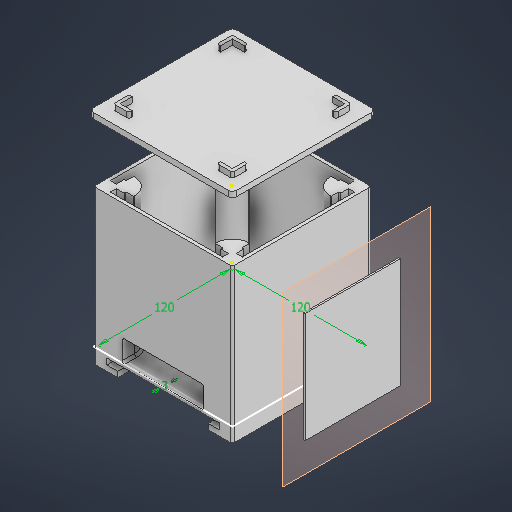
# Autodesk Inventor part: Chink_Box_FINAL
Saved by Autodesk Inventor 2026.1 (Build 301233020, 233B)
## iProperties
Created: 2026-09-22
Part Number: Chink_Box_FINAL
Material: Generic
Document SubType Name: Modeling
Designer: uali517
Density: 1 g/cm^3
Appearance: Default
Author: uali517
Autodesk Inventor part; units mm, degrees
ref_plane "YZ Plane" through (0, 0, 0) normal (1, 0, 0) x (0, 1, 0)
ref_plane "XY Plane" through (0, 0, 0) normal (0, 0, 1) x (1, 0, 0)
sketch "Sketch1" plane through (0, 0, 0) normal (0, 1, 0) x (-1, 0, 0)
  line L0 (0, 0) -> (120, 0)
  line L1 (120, 0) -> (120, -120)
  line L2 (120, -120) -> (0, -120)
  line L3 (0, -120) -> (0, 0)
  line L4 (123, 3) -> (-3, 3)
  line L5 (-3, 3) -> (-3, -123)
  line L6 (-3, -123) -> (123, -123)
  line L7 (123, -123) -> (123, 3)
  dimension "d0" = 120
  dimension "d1" = 120
  dimension "d2" = 3
  constraints: 16 end point, 4 parallel, 2 perpendicular, 1 horizontal, 3 other
  measures "d0" distance of L1.end L2.end
  measures "d1" distance of L0.end L1.end
  measures "d2" distance between parallel lines of L0 L4
extrude "Extrusion1" add sketch "Sketch1" along normal blind 126
sketch "Sketch2" plane through (0, 0, 0) normal (0, 1, 0) x (-1, 0, 0)
  line L0 (0, 0) -> (120, 0) projected
  line L1 (120, 0) -> (111, 0)
  line L2 (111, 0) -> (111, -9)
  line L3 (111, -9) -> (120, -9)
  line L4 (120, -9) -> (120, 0)
  line L5 (114.5, -5.5) -> (104, -5.5)
  line L6 (114.5, -16) -> (114.5, -5.5)
  line L7 (104, -5.5) -> (104, -16)
  line L8 (104, -16) -> (114.5, -16)
  line L9 (104, -7.3) -> (97, -7.3)
  line L10 (104, -13.4046) -> (104, -7.3)
  line L11 (112.7, -16) -> (106.6771, -16)
  line L12 (112.7, -23) -> (112.7, -16)
  line L13 (97, -7.3) -> (97, -8)
  line L14 (112, -23) -> (112.7, -23)
  arc A0 (97, -8) -> (112, -23) centre (112, -8) ccw
  point P0 (120, -120)
  point P1 (111, 0)
  point P2 (60, -60)
  point P3 (114.5, -9)
  point P4 (111, -5.5)
  dimension "d9" = 9
  dimension "d10" = 9
  dimension "d15" = 5.5
  dimension "d37" = 1.8
  dimension "d39" = 1.8
  dimension "d40" = 15
  dimension "d41" = 7
  dimension "d42" = 7
  constraints: 28 end point, 5 perpendicular, 4 horizontal, 2 parallel, 2 point on circle, 2 point on line, 2 tangent, 2 vertical, 1 centre point
  measures "d9" distance of L3.end L2.end
  measures "d10" distance of L2.end L1.end
  measures "d15" distance between parallel lines of L0 L5
  measures "d37" distance between parallel lines of L5 L9
  measures "d39" distance between parallel lines of L6 L12
  measures "d40" radius of A0
  measures "d41" distance of L9.start L9.end
  measures "d42" distance between parallel lines of L7 L2
extrude "Extrusion3" add sketch "Sketch2" along normal up to surface (126 mm away)
pattern_circular "Circular Pattern1" count 4 over 360 about axis through (-60, 0, -60) along (0, 1, 0) of "Extrusion3"
sketch "Sketch9" plane through (0, 0, 0) normal (0, 1, 0) x (-1, 0, 0)
  line L0 (97, -7.3) -> (104, -7.3) projected
  line L1 (104, -7.3) -> (104, -5.5) projected
  line L2 (104, -5.5) -> (111, -5.5) projected
  line L3 (111, -5.5) -> (111, 0) projected
  line L4 (114.5, -9) -> (114.5, -16) projected
  line L5 (112.7, -16) -> (112.7, -23) projected
  line L6 (120, -9) -> (114.5, -9) projected
  line L7 (112.7, -97) -> (112.7, -104) projected
  line L8 (112.7, -104) -> (114.5, -104) projected
  line L9 (114.5, -104) -> (114.5, -111) projected
  line L10 (114.5, -111) -> (120, -111) projected
  line L11 (9, 0) -> (9, -5.5) projected
  line L12 (9, -5.5) -> (16, -5.5) projected
  line L13 (16, -5.5) -> (16, -7.3) projected
  line L14 (16, -7.3) -> (23, -7.3) projected
  line L15 (9, 0) -> (111, 0) projected
  line L16 (120, -9) -> (120, -111) projected
  line L17 (23, -7.3) -> (23, 0)
  line L18 (97, -7.3) -> (97, 0)
  line L19 (112.7, -97) -> (120, -97)
  line L20 (112.7, -23) -> (120, -23)
  line L21 (114.5, -16) -> (112.7, -16) projected
  point P0 (0, 0)
  constraints: 8 end point, 4 point on line, 3 perpendicular, 1 vertical
extrude "Extrusion8" add sketch "Sketch9" along normal blind 20
sketch "Sketch10" plane through (-123, 0, 3) normal (0, 0, 1) x (1, 0, 0)
  line L0 (19, 20) -> (26, 20) projected
  line L1 (100, 0) -> (100, 126) projected
  line L2 (26, 20) -> (100, 20)
  line L3 (100, 20) -> (100, 0)
  line L4 (100, 0) -> (26, 0)
  line L5 (26, 0) -> (26, 20)
  point P0 (123, 0)
  constraints: 8 end point, 2 parallel, 1 horizontal, 1 perpendicular
extrude "Extrusion9" cut sketch "Sketch10" against normal blind 20
sketch "Sketch11" plane through (-123, 0, -123) normal (-1, 0, 0) x (0, 0, 1)
  line L0 (100, 20) -> (107, 20) projected
  line L1 (26, 0) -> (26, 126) projected
  line L2 (100, 20) -> (26, 20)
  line L3 (26, 20) -> (26, 0)
  line L4 (26, 0) -> (100, 0)
  line L5 (100, 0) -> (100, 20)
  point P0 (123, 0)
  point P1 (26, 20)
  constraints: 8 end point, 2 parallel, 1 horizontal, 1 perpendicular
extrude "Extrusion10" cut sketch "Sketch11" against normal blind 20
sketch "Sketch12" plane through (0, 0, 0) normal (0, -1, 0) x (1, 0, 0)
  line L0 (3, 3) -> (3, -123) projected
  line L1 (3, -123) -> (-123, -123) projected
  line L2 (3, 3) -> (-123, 3)
  line L3 (-123, 3) -> (-123, -123)
  line L4 (-123, -123) -> (3, -123)
  line L5 (3, -123) -> (3, 3)
  point P0 (0, 0)
  constraints: 8 end point, 2 parallel, 1 horizontal, 1 perpendicular
extrude "Extrusion11" add sketch "Sketch12" along normal blind 3
sketch "Sketch3" plane through (0, 0, 0) normal (0, 1, 0) x (-1, 0, 0)
  arc A0 (106.679, -5.5) -> (114.5, -13.321) centre (114.6771, -5.3229) ccw projected
  line L0 (111, 0) -> (106.679, 0)
  line L1 (106.679, 0) -> (106.679, -5.5)
  line L2 (106.679, -5.5) -> (111, -5.5)
  line L3 (111, -5.5) -> (111, 0)
  line L4 (114.5, -16) -> (114.5, -9) projected
  line L5 (120, -9) -> (120, -111) projected
  line L6 (114.5, -13.321) -> (120, -13.321)
  line L7 (120, -13.321) -> (120, -9)
  line L8 (120, -9) -> (114.5, -9)
  line L9 (114.5, -9) -> (114.5, -13.321)
  line L10 (9, 0) -> (111, 0) projected
  line L11 (13.321, -5.5) -> (9, -5.5)
  line L12 (9, -5.5) -> (9, 0)
  line L13 (9, 0) -> (13.321, 0)
  line L14 (13.321, 0) -> (13.321, -5.5)
  line L15 (114.5, -111) -> (120, -111)
  line L16 (120, -111) -> (120, -106.679)
  line L17 (120, -106.679) -> (114.5, -106.679)
  line L18 (114.5, -106.679) -> (114.5, -111)
  point P0 (0, 0)
  constraints: 32 end point, 8 parallel, 4 horizontal, 4 perpendicular, 1 point on line
extrude "Extrusion4" [suppressed]
sketch "Sketch4" plane through (-120, 126, -9) normal (1, 0, 0) x (0, 0, -1)
  line L0 (97.679, -100) -> (97.679, -80) projected
  line L1 (4.321, -100) -> (4.321, -80) projected
  line L2 (97.679, -100) -> (97.679, -80) projected
  line L3 (97.679, -80) -> (4.321, -80)
  line L4 (4.321, -80) -> (4.321, -100)
  line L5 (4.321, -100) -> (97.679, -100)
  line L6 (97.679, -100) -> (97.679, -80)
  point P0 (-9, -126)
  point P1 (4.321, -80)
  constraints: 8 end point, 2 parallel, 1 horizontal, 1 perpendicular
extrude "Extrusion5" [suppressed]
sketch "Sketch5" plane through (-125, 0, 5) normal (0, 0, 1) x (1, 0, 0)
  line L0 (18.321, 20) -> (18.321, 100) projected
  line L1 (111.679, 0) -> (111.679, 100) projected
  line L2 (18.321, 20) -> (111.679, 20)
  line L3 (111.679, 20) -> (111.679, 0)
  line L4 (111.679, 0) -> (18.321, 0)
  line L5 (18.321, 0) -> (18.321, 20)
  point P0 (125, 0)
  constraints: 8 end point, 2 parallel, 1 horizontal, 1 perpendicular
extrude "Extrusion6" [suppressed]
sketch "Sketch6" plane through (0, 0, 0) normal (0, -1, 0) x (1, 0, 0)
  line L0 (5, 5) -> (5, -125) projected
  line L1 (-125, -13.321) -> (-125, 5) projected
  line L2 (5, -125) -> (-125, -125)
  line L3 (-125, -125) -> (-125, 5)
  line L4 (-125, 5) -> (5, 5)
  line L5 (5, 5) -> (5, -125)
  point P0 (0, 0)
  constraints: 8 end point, 2 parallel, 1 horizontal, 1 perpendicular
extrude "Extrusion7" [suppressed]
sketch "Sketch7" plane through (0, -5, 0) normal (0, -1, 0) x (1, 0, 0)
  point P0 (0, 0)
sketch "Sketch13" plane through (-123, 126, 3) normal (0, 0, 1) x (1, 0, 0)
  line L0 (0, -129) -> (126, -129) projected
  line L1 (126, -129) -> (126, -139.5)
  line L2 (126, -139.5) -> (104, -139.5)
  line L3 (104, -139.5) -> (104, -134.5)
  line L4 (104, -134.5) -> (114, -134.5)
  line L5 (114, -134.5) -> (114, -129)
  point P0 (123, -126)
  dimension "d51" = 12
  dimension "d52" = 5.5
  dimension "d53" = 5
  dimension "d56" = 10
  constraints: 10 end point, 4 perpendicular, 1 point on line, 1 vertical
  measures "d51" distance between parallel lines of L1 L5
  measures "d52" distance between parallel lines of L0 L4
  measures "d53" distance between parallel lines of L4 L2
  measures "d56" distance of L3.end L4.end
sketch3d "3D Sketch2"
  line L0 (3, -3, 3) -> (3, -3, -123)
  line L1 (3, -3, -123) -> (-123, -3, -123)
  line L2 (-123, -3, -123) -> (-123, -3, 3)
sweep "Sweep2" add profiles "Sketch13" path "3D Sketch2"
fillet "Fillet1" radius 2 4 edges at (3, 56.25, 3) (3, 56.25, -123) (-123, 56.25, 3) (-123, 56.25, -123)
fillet "Fillet2" radius 2 9 edges at (-97, 20, 1.5) (-97, 20, -3.65) (-23, 20, 1.5) (-23, 20, -3.65) (-101.3934, 0, -18.6066) (-18.6066, 0, -18.6066) (-7.65, 0, -23) (-97, 0, -112.35) (-101.3934, 0, -101.3934)
sketch "Sketch14" plane through (-120, 126, -9) normal (1, 0, 0) x (0, 0, -1)
  point P0 (-9, -126)
sketch "Sketch15" plane through (0, 126, 0) normal (0, 1, 0) x (1, 0, 0)
  point P0 (0, 0)
ref_plane "Work Plane1" through (0, 176, 0) normal (0, 1, 0) x (1, 0, 0)
sketch "Sketch16" plane through (0, 176, 0) normal (0, 1, 0) x (1, 0, 0)
  arc A0 (-121, 123) -> (-123, 121) centre (-121, 121) ccw projected
  line L0 (-123, 121) -> (-123, -1) projected
  arc A1 (-123, -1) -> (-121, -3) centre (-121, -1) ccw projected
  line L1 (-121, -3) -> (1, -3) projected
  arc A2 (1, -3) -> (3, -1) centre (1, -1) ccw projected
  line L2 (3, -1) -> (3, 121) projected
  arc A3 (3, 121) -> (1, 123) centre (1, 121) ccw projected
  line L3 (1, 123) -> (-121, 123) projected
  line L4 (-9, 0) -> (-111, 0) projected
  line L5 (-111, 5.5) -> (-111, 0) projected
  line L6 (-104, 5.5) -> (-111, 5.5) projected
  line L7 (-104, 7.3) -> (-104, 5.5) projected
  line L8 (-97, 7.3) -> (-104, 7.3) projected
  line L9 (-97, 8) -> (-97, 7.3) projected
  arc A4 (-97, 8) -> (-112, 23) centre (-112, 8) ccw projected
  line L10 (-112.7, 23) -> (-112, 23) projected
  line L11 (-112.7, 16) -> (-112.7, 23) projected
  line L12 (-114.5, 16) -> (-112.7, 16) projected
  line L13 (-114.5, 9) -> (-114.5, 16) projected
  line L14 (-120, 9) -> (-114.5, 9) projected
  line L15 (-120, 9) -> (-120, 111) projected
  line L16 (-114.5, 111) -> (-120, 111) projected
  line L17 (-114.5, 104) -> (-114.5, 111) projected
  line L18 (-112.7, 104) -> (-114.5, 104) projected
  line L19 (-112.7, 97) -> (-112.7, 104) projected
  line L20 (-112, 97) -> (-112.7, 97) projected
  arc A5 (-112, 97) -> (-97, 112) centre (-112, 112) ccw projected
  line L21 (-97, 112.7) -> (-97, 112) projected
  line L22 (-104, 112.7) -> (-97, 112.7) projected
  line L23 (-104, 114.5) -> (-104, 112.7) projected
  line L24 (-111, 114.5) -> (-104, 114.5) projected
  line L25 (-111, 120) -> (-111, 114.5) projected
  line L26 (-111, 120) -> (-9, 120) projected
  line L27 (-9, 114.5) -> (-9, 120) projected
  line L28 (-16, 114.5) -> (-9, 114.5) projected
  line L29 (-16, 112.7) -> (-16, 114.5) projected
  line L30 (-23, 112.7) -> (-16, 112.7) projected
  line L31 (-23, 112) -> (-23, 112.7) projected
  arc A6 (-23, 112) -> (-8, 97) centre (-8, 112) ccw projected
  line L32 (-7.3, 97) -> (-8, 97) projected
  line L33 (-7.3, 104) -> (-7.3, 97) projected
  line L34 (-5.5, 104) -> (-7.3, 104) projected
  line L35 (-5.5, 111) -> (-5.5, 104) projected
  line L36 (0, 111) -> (-5.5, 111) projected
  line L37 (0, 111) -> (0, 9) projected
  line L38 (-5.5, 9) -> (0, 9) projected
  line L39 (-5.5, 16) -> (-5.5, 9) projected
  line L40 (-7.3, 16) -> (-5.5, 16) projected
  line L41 (-7.3, 23) -> (-7.3, 16) projected
  line L42 (-8, 23) -> (-7.3, 23) projected
  arc A7 (-8, 23) -> (-23, 8) centre (-8, 8) ccw projected
  line L43 (-23, 7.3) -> (-23, 8) projected
  line L44 (-16, 7.3) -> (-23, 7.3) projected
  line L45 (-16, 5.5) -> (-16, 7.3) projected
  line L46 (-9, 5.5) -> (-16, 5.5) projected
  line L47 (-9, 0) -> (-9, 5.5) projected
  line L48 (-109.5, 1.5) -> (-10.5, 1.5)
  line L49 (-10.5, 1.5) -> (-10.5, 4)
  line L50 (-10.5, 4) -> (-17.5, 4)
  line L51 (-17.5, 4) -> (-17.5, 5.8)
  line L52 (-17.5, 5.8) -> (-24.5, 5.8)
  line L53 (-24.5, 5.8) -> (-24.5, 8)
  arc A8 (-8, 24.5) -> (-24.5, 8) centre (-8, 8) ccw
  line L54 (-8, 24.5) -> (-5.8, 24.5)
  line L55 (-5.8, 24.5) -> (-5.8, 17.5)
  line L56 (-5.8, 17.5) -> (-4, 17.5)
  line L57 (-4, 17.5) -> (-4, 10.5)
  line L58 (-4, 10.5) -> (-1.5, 10.5)
  line L59 (-1.5, 10.5) -> (-1.5, 109.5)
  line L60 (-1.5, 109.5) -> (-4, 109.5)
  line L61 (-4, 109.5) -> (-4, 102.5)
  line L62 (-4, 102.5) -> (-5.8, 102.5)
  line L63 (-5.8, 102.5) -> (-5.8, 95.5)
  line L64 (-5.8, 95.5) -> (-8, 95.5)
  arc A9 (-24.5, 112) -> (-8, 95.5) centre (-8, 112) ccw
  line L65 (-24.5, 112) -> (-24.5, 114.2)
  line L66 (-24.5, 114.2) -> (-17.5, 114.2)
  line L67 (-17.5, 114.2) -> (-17.5, 116)
  line L68 (-17.5, 116) -> (-10.5, 116)
  line L69 (-10.5, 116) -> (-10.5, 118.5)
  line L70 (-10.5, 118.5) -> (-109.5, 118.5)
  line L71 (-109.5, 118.5) -> (-109.5, 116)
  line L72 (-109.5, 116) -> (-102.5, 116)
  line L73 (-102.5, 116) -> (-102.5, 114.2)
  line L74 (-102.5, 114.2) -> (-95.5, 114.2)
  line L75 (-95.5, 114.2) -> (-95.5, 112)
  arc A10 (-112, 95.5) -> (-95.5, 112) centre (-112, 112) ccw
  line L76 (-112, 95.5) -> (-114.2, 95.5)
  line L77 (-114.2, 95.5) -> (-114.2, 102.5)
  line L78 (-114.2, 102.5) -> (-116, 102.5)
  line L79 (-116, 102.5) -> (-116, 109.5)
  line L80 (-116, 109.5) -> (-118.5, 109.5)
  line L81 (-118.5, 109.5) -> (-118.5, 10.5)
  line L82 (-118.5, 10.5) -> (-116, 10.5)
  line L83 (-116, 10.5) -> (-116, 17.5)
  line L84 (-116, 17.5) -> (-114.2, 17.5)
  line L85 (-114.2, 17.5) -> (-114.2, 24.5)
  line L86 (-114.2, 24.5) -> (-112, 24.5)
  arc A11 (-95.5, 8) -> (-112, 24.5) centre (-112, 8) ccw
  line L87 (-95.5, 8) -> (-95.5, 5.8)
  line L88 (-95.5, 5.8) -> (-102.5, 5.8)
  line L89 (-102.5, 5.8) -> (-102.5, 4)
  line L90 (-102.5, 4) -> (-109.5, 4)
  line L91 (-109.5, 4) -> (-109.5, 1.5)
  point P0 (0, 0)
  dimension "d60" = 1.5
  constraints: 88 end point, 8 point on circle, 4 centre point, 47 other
  measures "d60" distance between parallel lines of L4 L48
extrude "Extrusion12" add sketch "Sketch16" along normal blind 5 separate body contours L91 L90 L89 L88 L87 A11 L86 L85 L84 L83 L82 L81 L80 L79 L78 L77 L76 A10 L75 L74 L73 L72 L71 L70 L69 L68 L67 L66 L65 A9 L64 L63 L62 L61 L60 L59 L58 L57 L56 L55 L54 A8 L53 L52 L51 L50 L49 L48
sketch "Sketch17" plane through (0, 181, 0) normal (0, 1, 0) x (1, 0, 0)
  arc A0 (-121, 123) -> (-123, 121) centre (-121, 121) ccw projected
  line L0 (-123, 121) -> (-123, -1) projected
  arc A1 (-123, -1) -> (-121, -3) centre (-121, -1) ccw projected
  line L1 (-121, -3) -> (1, -3) projected
  arc A2 (1, -3) -> (3, -1) centre (1, -1) ccw projected
  line L2 (3, -1) -> (3, 121) projected
  arc A3 (3, 121) -> (1, 123) centre (1, 121) ccw projected
  line L3 (1, 123) -> (-121, 123) projected
  line L4 (-9, 0) -> (-111, 0) projected
  line L5 (-111, 5.5) -> (-111, 0) projected
  line L6 (-104, 5.5) -> (-111, 5.5) projected
  line L7 (-104, 7.3) -> (-104, 5.5) projected
  line L8 (-97, 7.3) -> (-104, 7.3) projected
  line L9 (-97, 8) -> (-97, 7.3) projected
  arc A4 (-97, 8) -> (-112, 23) centre (-112, 8) ccw projected
  line L10 (-112.7, 23) -> (-112, 23) projected
  line L11 (-112.7, 16) -> (-112.7, 23) projected
  line L12 (-114.5, 16) -> (-112.7, 16) projected
  line L13 (-114.5, 9) -> (-114.5, 16) projected
  line L14 (-120, 9) -> (-114.5, 9) projected
  line L15 (-120, 9) -> (-120, 111) projected
  line L16 (-114.5, 111) -> (-120, 111) projected
  line L17 (-114.5, 104) -> (-114.5, 111) projected
  line L18 (-112.7, 104) -> (-114.5, 104) projected
  line L19 (-112.7, 97) -> (-112.7, 104) projected
  line L20 (-112, 97) -> (-112.7, 97) projected
  arc A5 (-112, 97) -> (-97, 112) centre (-112, 112) ccw projected
  line L21 (-97, 112.7) -> (-97, 112) projected
  line L22 (-104, 112.7) -> (-97, 112.7) projected
  line L23 (-104, 114.5) -> (-104, 112.7) projected
  line L24 (-111, 114.5) -> (-104, 114.5) projected
  line L25 (-111, 120) -> (-111, 114.5) projected
  line L26 (-111, 120) -> (-9, 120) projected
  line L27 (-9, 114.5) -> (-9, 120) projected
  line L28 (-16, 114.5) -> (-9, 114.5) projected
  line L29 (-16, 112.7) -> (-16, 114.5) projected
  line L30 (-23, 112.7) -> (-16, 112.7) projected
  line L31 (-23, 112) -> (-23, 112.7) projected
  arc A6 (-23, 112) -> (-8, 97) centre (-8, 112) ccw projected
  line L32 (-7.3, 97) -> (-8, 97) projected
  line L33 (-7.3, 104) -> (-7.3, 97) projected
  line L34 (-5.5, 104) -> (-7.3, 104) projected
  line L35 (-5.5, 111) -> (-5.5, 104) projected
  line L36 (0, 111) -> (-5.5, 111) projected
  line L37 (0, 111) -> (0, 9) projected
  line L38 (-5.5, 9) -> (0, 9) projected
  line L39 (-5.5, 16) -> (-5.5, 9) projected
  line L40 (-7.3, 16) -> (-5.5, 16) projected
  line L41 (-7.3, 23) -> (-7.3, 16) projected
  line L42 (-8, 23) -> (-7.3, 23) projected
  arc A7 (-8, 23) -> (-23, 8) centre (-8, 8) ccw projected
  line L43 (-23, 7.3) -> (-23, 8) projected
  line L44 (-16, 7.3) -> (-23, 7.3) projected
  line L45 (-16, 5.5) -> (-16, 7.3) projected
  line L46 (-9, 5.5) -> (-16, 5.5) projected
  line L47 (-9, 0) -> (-9, 5.5) projected
  line L48 (1, -5) -> (-121, -5)
  arc A8 (-125, -1) -> (-121, -5) centre (-121, -1) ccw
  line L49 (-125, -1) -> (-125, 121)
  arc A9 (-121, 125) -> (-125, 121) centre (-121, 121) ccw
  line L50 (-121, 125) -> (1, 125)
  arc A10 (5, 121) -> (1, 125) centre (1, 121) ccw
  line L51 (5, 121) -> (5, -1)
  arc A11 (1, -5) -> (5, -1) centre (1, -1) ccw
  point P0 (0, 0)
  dimension "d63" = 2
  constraints: 8 end point, 8 point on circle, 4 centre point, 7 other
  measures "d63" distance between parallel lines of L1 L48
extrude "Extrusion13" add sketch "Sketch17" along normal blind 5 contours L3 A3 L2 A2 L1 A1 L0 A0 | L4 L5 L6 L7 L8 L9 A4 L10 L11 L12 L13 L14 L15 L16 L17 L18 L19 L20 A5 L21 L22 L23 L24 L25 L26 L27 L28 L29 L30 L31 A6 L32 L33 L34 L35 L36 L37 L38 L39 L40 L41 L42 A7 L43 L44 L45 L46 L47 | L48 A8 L49 A9 L50 A10 L51 A11 bodies 2
sketch "Sketch18" plane through (0, 186, 0) normal (0, 1, 0) x (1, 0, 0)
  point P0 (0, 0)
sketch "Sketch19" plane through (0, 186, 0) normal (0, 1, 0) x (1, 0, 0)
  line L0 (1, 125) -> (-121, 125) projected
  arc A0 (-121, 125) -> (-125, 121) centre (-121, 121) ccw projected
  line L1 (-125, 121) -> (-125, -1) projected
  arc A1 (-125, -1) -> (-121, -5) centre (-121, -1) ccw projected
  line L2 (-121, -5) -> (1, -5) projected
  arc A2 (1, -5) -> (5, -1) centre (1, -1) ccw projected
  line L3 (5, -1) -> (5, 121) projected
  arc A3 (5, 121) -> (1, 125) centre (1, 121) ccw projected
  line L4 (-9, 9) -> (-111, 9)
  line L5 (-111, 9) -> (-111, 111)
  line L6 (-111, 111) -> (-9, 111)
  line L7 (-9, 111) -> (-9, 9)
  line L8 (-60, 60) -> (-60, 50.9417)
  line L9 (-60, 60) -> (-68.1183, 60)
  line L10 (-6, 6) -> (-114, 6)
  line L11 (-114, 6) -> (-114, 114)
  line L12 (-114, 114) -> (-6, 114)
  line L13 (-6, 114) -> (-6, 6)
  line L14 (-100, 9) -> (-20, 9)
  line L15 (-20, 9) -> (-20, 6)
  line L16 (-20, 6) -> (-100, 6)
  line L17 (-100, 6) -> (-100, 9)
  line L18 (-20, 111) -> (-100, 111)
  line L19 (-100, 111) -> (-100, 114)
  line L20 (-100, 114) -> (-20, 114)
  line L21 (-20, 114) -> (-20, 111)
  line L22 (-111, 20) -> (-114, 20)
  line L23 (-114, 20) -> (-114, 100)
  line L24 (-114, 100) -> (-111, 100)
  line L25 (-111, 100) -> (-111, 20)
  line L26 (-6, 20) -> (-9, 20)
  line L27 (-9, 20) -> (-9, 100)
  line L28 (-9, 100) -> (-6, 100)
  line L29 (-6, 100) -> (-6, 20)
  point P0 (0, 0)
  point P1 (-100, 7.5)
  point P2 (-20, 7.5)
  point P3 (-100, 6)
  point P4 (-20, 9)
  point P5 (-6, 100)
  dimension "d66" = 102
  dimension "d67" = 102
  dimension "d68" = 3
  dimension "d69" = 80
  dimension "d70" = 80
  dimension "d71" = 80
  constraints: 52 end point, 12 parallel, 8 point on line, 6 horizontal, 6 perpendicular, 2 midpoint, 1 vertical, 9 other
  measures "d66" distance of L5.end L6.end
  measures "d67" distance of L4.end L5.end
  measures "d68" distance between parallel lines of L7 L13
  measures "d69" distance of point (-100, 7.5) point (-20, 7.5)
  measures "d70" distance of L22.end L23.end
  measures "d71" distance between parallel lines of L19 L21
extrude "Extrusion14" add sketch "Sketch19" along normal blind 5 contours L7 L26 L13 L10 L15 L4 | L17 L10 L11 L22 L5 L4 | L7 L6 L21 L12 L13 L28 | L24 L11 L12 L19 L6 L5 bodies 2
fillet "Fillet3" radius 2 12 edges at (-6, 188.5, -6) (-114, 188.5, -6) (-114, 188.5, -114) (-6, 188.5, -114) (-100, 188.5, -114) (-114, 188.5, -100) (-20, 188.5, -114) (-6, 188.5, -100) (-6, 188.5, -20) (-20, 188.5, -6) (-100, 188.5, -6) (-114, 188.5, -20)
ref_plane "Work Plane2" through (53, -13.5, -121) normal (1, 0, 0) x (0, 0, -1)
sketch "Sketch20" plane through (53, -13.5, -121) normal (1, 0, 0) x (0, 0, -1)
  line L0 (-109.3671, 20.8626) -> (-22.8671, 20.8626)
  line L1 (-22.8671, 20.8626) -> (-22.8671, 120.8626)
  line L2 (-22.8671, 120.8626) -> (-109.3671, 120.8626)
  line L3 (-109.3671, 120.8626) -> (-109.3671, 20.8626)
  point P0 (-121, 13.5)
  dimension "d76" = 86.5
  dimension "d77" = 100
  constraints: 8 end point, 2 parallel, 1 horizontal, 1 perpendicular
  measures "d76" distance of L2.end L1.end
  measures "d77" distance of L1.end L0.end
extrude "Extrusion15" add sketch "Sketch20" along normal blind 1.5 separate body
sketch "Sketch8" plane through (3, 126, 3) normal (1, 0, 0) x (0, 0, -1)
  line L0 (0, -105) -> (130, -105) projected
  line L1 (14, -105) -> (14, -110.5)
  line L2 (0, 0) -> (0, -105) projected
  line L3 (0, -105) -> (0, -115.5)
  line L4 (0, -115.5) -> (19, -115.5)
  line L5 (19, -115.5) -> (19, -110.5)
  line L6 (19, -110.5) -> (14, -110.5)
  point P0 (3, -126)
  dimension "d31" = 14
  dimension "d32" = 5.5
  dimension "d33" = 5
  constraints: 10 end point, 4 perpendicular, 2 vertical, 1 point on line
  measures "d31" distance between parallel lines of L2 L1
  measures "d32" distance from line of L0 L1.end
  measures "d33" distance of L5.end L1.end
sketch3d "3D Sketch1"
